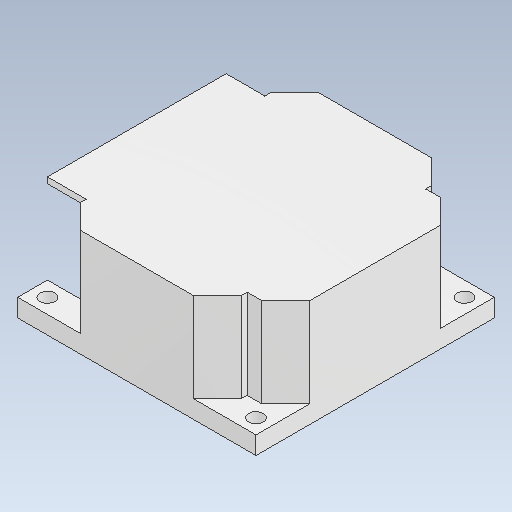
# Autodesk Inventor part: obudowa_gps_bt
Saved by Autodesk Inventor 2020 (Build 240168000, 168)
## iProperties
Created: 2020-08-30
Part Number: obudowa_gps_bt
Material: ABS Plastic
Document SubType Name: Modeling
Designer: Hesekiel
Density: 1.06 g/cm^3
Appearance: Smooth - White
Mass: 10.7461 g
Surface Area: 65.376 cm^2
Volume: 10.1379 cm^3
Author: Hesekiel
Autodesk Inventor part; units mm, degrees
ref_plane "YZ Plane" through (0, 0, 0) normal (1, 0, 0) x (0, 1, 0)
ref_plane "XZ Plane" through (0, 0, 0) normal (0, 1, 0) x (-1, 0, 0)
ref_plane "XY Plane" through (0, 0, 0) normal (0, 0, 1) x (1, 0, 0)
sketch "Sketch1" plane through (0, 0, 0) normal (0, 1, 0) x (-1, 0, 0)
  line L0 (-17.5, 17.5) -> (17.5, -17.5) construction
  line L1 (17.5, 17.5) -> (-17.5, -17.5) construction
  circle A0 centre (17.5, 17.5) radius 1.25
  circle A1 centre (-17.5, 17.5) radius 1.25
  circle A2 centre (17.5, -17.5) radius 1.25
  circle A3 centre (-17.5, -17.5) radius 1.25
  line L2 (-20, 20) -> (20, 20)
  line L3 (20, 20) -> (20, -20)
  line L4 (20, -20) -> (-20, -20)
  line L5 (-20, -20) -> (-20, 20)
  line L6 (-20, 20) -> (20, -20) construction
  line L7 (20, 20) -> (-20, -20) construction
  point P0 (0, 0)
  dimension "d0" = 35
  dimension "d1" = 35
  dimension "d2" = 2.5
  dimension "d3" = 2.5
  dimension "d4" = 2.5
  dimension "d5" = 2.5
  dimension "d6" = 40
  dimension "d7" = 40
  constraints: 16 end point, 4 centre point, 4 coincident, 4 midpoint, 2 parallel, 1 horizontal, 1 perpendicular
  measures "d0" distance of L0.end L1.end
  measures "d1" distance of L1.start L0.end
  measures "d2" diameter of A0
  measures "d3" diameter of A1
  measures "d4" diameter of A2
  measures "d5" diameter of A3
  measures "d6" distance of L3.end L4.end
  measures "d7" distance of L2.end L3.end
extrude "Extrusion2" add sketch "Sketch1" along normal blind 3
sketch "Sketch2" plane through (0, 3, 0) normal (0, 1, 0) x (1, 0, 0)
  line L0 (20, -15) -> (-20, -15)
  line L1 (-20, -15) -> (-20, 15)
  line L2 (-20, 15) -> (20, 15)
  line L3 (20, 15) -> (20, -15)
  line L4 (20, -15) -> (-20, 15) construction
  line L5 (-20, -15) -> (20, 15) construction
  line L6 (-13.5, 10) -> (13.5, 10)
  line L7 (13.5, 10) -> (13.5, 20)
  line L8 (13.5, 20) -> (-13.5, 20)
  line L9 (-13.5, 20) -> (-13.5, 10)
  line L10 (-13.5, 10) -> (13.5, 20) construction
  line L11 (13.5, 10) -> (-13.5, 20) construction
  line L12 (-13.5, -10) -> (13.5, -10)
  line L13 (13.5, -10) -> (13.5, -20)
  line L14 (13.5, -20) -> (-13.5, -20)
  line L15 (-13.5, -20) -> (-13.5, -10)
  line L16 (-13.5, -10) -> (13.5, -20) construction
  line L17 (13.5, -10) -> (-13.5, -20) construction
  point P0 (0, 0)
  point P1 (0, 15)
  point P2 (0, -15)
  point P3 (13.5, -15)
  point P4 (-13.5, -15)
  point P5 (-13.5, 15)
  point P6 (13.5, 15)
  dimension "d12" = 40
  dimension "d13" = 30
  dimension "d27" = 27
  dimension "d28" = 10
  dimension "d29" = 27
  dimension "d30" = 10
  constraints: 36 end point, 8 midpoint, 6 parallel, 3 horizontal, 3 perpendicular
  measures "d12" distance of L1.end L2.end
  measures "d13" distance of L0.end L1.end
  measures "d27" distance of L8.end L7.end
  measures "d28" distance of L7.end L6.end
  measures "d29" distance of L13.end L14.end
  measures "d30" distance of L12.end L13.end
extrude "Extrusion3" add sketch "Sketch2" along normal blind 15
sketch "Sketch4" plane through (-20, 0, -20) normal (-1, 0, 0) x (0, 0, 1)
  line L0 (0, 0) -> (40, 0) projected
  line L1 (40, 0) -> (40, 3) projected
  line L2 (35, 3) -> (40, 3) projected
  line L3 (35, 3) -> (35, 18) projected
  line L4 (5, 18) -> (35, 18) projected
  line L5 (5, 3) -> (5, 18) projected
  line L6 (0, 3) -> (5, 3) projected
  line L7 (0, 0) -> (0, 3) projected
  line L8 (33.5, -17) -> (6.5, -17)
  line L9 (6.5, -17) -> (6.5, 17)
  line L10 (6.5, 17) -> (33.5, 17)
  line L11 (33.5, 17) -> (33.5, -17)
  line L12 (33.5, -17) -> (6.5, 17) construction
  line L13 (6.5, -17) -> (33.5, 17) construction
  line L14 (5, 18) -> (6.5, 18)
  line L15 (6.5, 18) -> (6.5, 0)
  line L16 (6.5, 0) -> (5, 0)
  line L17 (5, 0) -> (5, 18)
  line L18 (5, 18) -> (35, 18) projected
  line L19 (35, 18) -> (33.5, 18)
  line L20 (33.5, 18) -> (33.5, 0)
  line L21 (33.5, 0) -> (35, 0)
  line L22 (35, 0) -> (35, 18)
  line L23 (6.5, 17) -> (5, 17)
  line L24 (33.5, 17) -> (35, 17)
  point P0 (20, 0)
  dimension "d20" = 27
  dimension "d21" = 34
  constraints: 32 end point, 6 parallel, 4 midpoint, 4 perpendicular, 3 horizontal, 3 point on line
  measures "d20" distance of L9.end L10.end
  measures "d21" distance of L8.end L9.end
extrude "Extrusion5" cut sketch "Sketch4" against normal blind 31 contours L17 L5 L23 L9 L0 | L9 L10 L11 L0 | L11 L24 L3 L22 L0
chamfer "Chamfer2" distance 2 angle 45 2 edges at (-4.5, 0, -15) (-4.5, 0, 15)
chamfer "Chamfer3" distance 4 angle 45 6 edges at (20, 10.5, -15) (13.5, 10.5, -20) (-13.5, 10.5, -20) (-13.5, 10.5, 20) (13.5, 10.5, 20) (20, 10.5, 15)
body "Solid2"
